0.5Offset v3 (Autodesk Fusion 360 design; units mm, degrees)
Autodesk Fusion 360 part; units mm, degrees
sketch "Sketch1" plane through (0, 0, 0) normal (0, 1, 0) x (1, 0, 0)
  circle A0 centre (0, 0) radius 32.5
  circle A1 centre (0, 0) radius 28.5
  dimension "d1" = 65
  dimension "d2" = 57
  constraint coincident A0.centre A1.centre
  measures "d1" diameter of A0
  measures "d2" diameter of A1
extrude "Extrude1" add sketch "Sketch1" along normal blind 10 makes body 1
sketch "Sketch2" plane through (0, 10, 0) normal (0, 1, 0) x (-1, 0, 0)
  circle A0 centre (0, 0) radius 28.5
  circle A1 centre (0, 0) radius 32.5
  circle A2 centre (0, 0) radius 28.5
  circle A3 centre (0, 0) radius 28
  circle A4 centre (0, 0) radius 27
  dimension "d5" = -0.5
  dimension "d8" = -1.5
extrude "Extrude3" add sketch "Sketch2" along normal blind 30 and the other way blind 5 separate body contours A3 makes body 2
sketch "Sketch3" plane through (0, 0, 0) normal (0, -1, 0) x (1, 0, 0)
  circle A0 centre (0, 0) radius 28.5
  circle A1 centre (0, 0) radius 32.5
  circle A2 centre (0, 0) radius 28.5
  circle A3 centre (0, 0) radius 28
extrude "Extrude4" add sketch "Sketch3" against normal blind 10 contours A0 A2 bodies 1 2
fillet "Fillet1" radius 1 1 edges at (26.1052, 5, 10.1252) on bodies 1
chamfer "Chamfer1" distance 0.5 angle 45 1 edges at (26.1052, 40, -10.1252) on bodies 1 2
equation "d8 = -0.5 mm - 1 mm"
